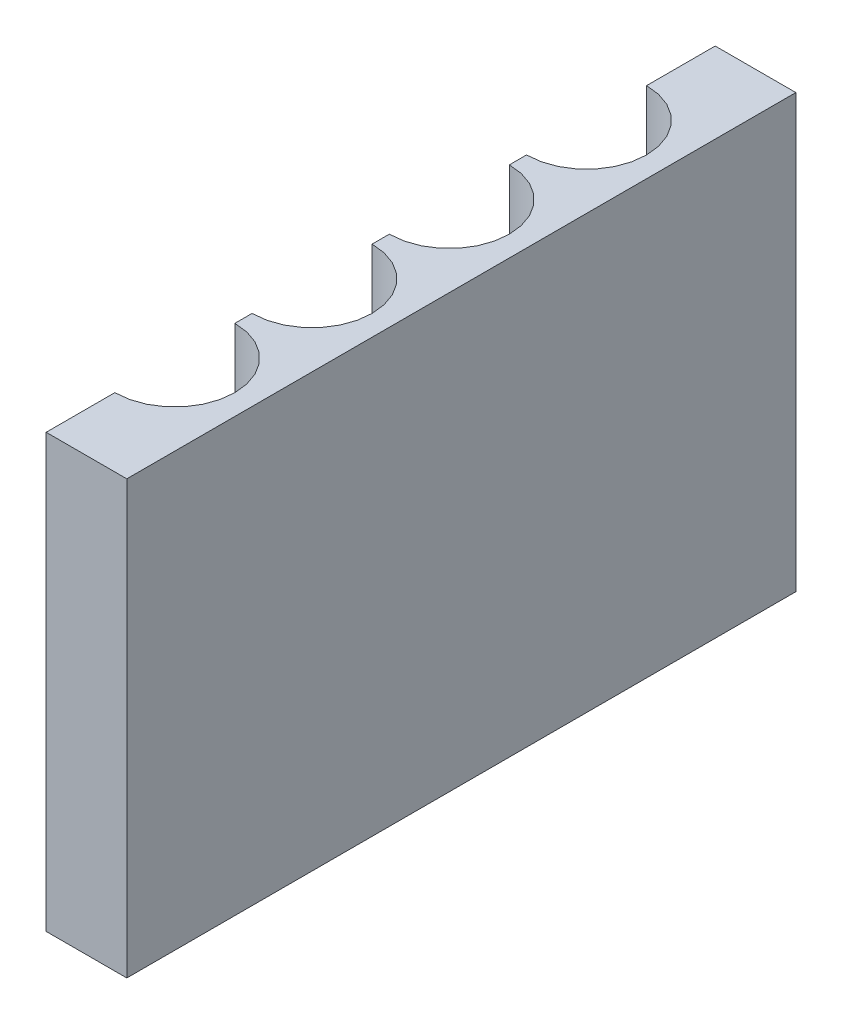
# Autodesk Inventor part: BatteryHolder
Saved by Autodesk Inventor 2023 (Build 270158000, 158)
## iProperties
Created: 2022-08-06
Part Number: BatteryHolder
Material: Generic
Document SubType Name: Modeling
Designer: Aditya Bansal
Density: 1 g/cm^3
Appearance: Default
Author: Aditya Bansal
Autodesk Inventor part; units mm, degrees
ref_plane "YZ Plane" through (0, 0, 0) normal (1, 0, 0) x (0, 1, 0)
ref_plane "XZ Plane" through (0, 0, 0) normal (0, 1, 0) x (-1, 0, 0)
ref_plane "XY Plane" through (0, 0, 0) normal (0, 0, 1) x (1, 0, 0)
sketch "Sketch1" plane through (0, 0, 0) normal (0, 1, 0) x (-1, 0, 0)
  line L0 (0, 0) -> (11.75, 0)
  line L1 (11.75, 0) -> (11.75, -97.5)
  line L2 (11.75, -97.5) -> (0, -97.5)
  line L3 (0, -97.5) -> (0, 0)
  circle A0 centre (11.75, -18.75) radius 8.75
  circle A1 centre (11.75, -38.75) radius 8.75
  circle A2 centre (11.75, -58.75) radius 8.75
  circle A3 centre (11.75, -78.75) radius 8.75
  point P0 (11.75, -87.5)
  point P1 (11.75, -70)
  point P2 (11.75, -67.5)
  point P3 (11.75, -50)
  point P4 (11.75, -47.5)
  point P5 (11.75, -30)
  point P6 (11.75, -27.5)
  point P7 (11.75, -10)
  dimension "d0" = 17.5
  dimension "d4" = 20
  dimension "d9" = 3
  dimension "d11" = 10
  dimension "d12" = 10
  constraints: 8 end point, 4 centre point, 2 parallel, 1 horizontal, 1 perpendicular, 1 point on line, 1 vertical, 6 other
  measures "d0" diameter of A0
  measures "d4" distance of A0.centre A1.centre
  measures "d9" distance edge to line of A3 L3
  measures "d11" distance edge to line of A3 L2
  measures "d12" distance edge to line of A0 L0
extrude "Extrusion1" add sketch "Sketch1" along normal blind 63 contours L0 L1 A0 A1 A2 A3 L2 L3
equation "\"d12\" = d11"
body "Solid1"
